Autodesk Fusion 360 part; units mm, degrees
(part 2 of 2)
sketch "Sketch10" plane through (0, 0, 0) normal (0, 0, 1) x (-1, 0, 0)
  line L0 (-14.3967, 6.981) -> (-3.4714, 1.9873)
  arc A0 (-3.4714, 1.9873) -> (-4, 0.0153) centre (0, 0) ccw
  line L1 (-4, 0.0153) -> (-12.1678, 3.0017)
  arc A1 (-14.3967, 6.981) -> (-12.1678, 3.0017) centre (-10.9658, 6.2889) ccw
  line L2 (-11.0881, -11.5349) -> (-2.9627, -2.6874)
  arc A2 (-2.9627, -2.6874) -> (-1.2506, -3.7995) centre (0, 0) ccw
  line L3 (-1.2506, -3.7995) -> (-6.6149, -10.6446)
  arc A3 (-11.0881, -11.5349) -> (-6.6149, -10.6446) centre (-9.3697, -8.4858) ccw
  line L4 (2.1904, 15.8494) -> (0.8173, 3.9156)
  arc A4 (0.8173, 3.9156) -> (-1.2215, 3.8089) centre (0, 0) ccw
  line L5 (-1.2215, 3.8089) -> (-0.9052, 12.4998)
  arc A5 (2.1904, 15.8494) -> (-0.9052, 12.4998) centre (2.5925, 12.3725) ccw
  line L6 (7.5439, -14.1099) -> (1.6404, -3.6482)
  arc A6 (1.6404, -3.6482) -> (3.2271, -2.3635) centre (0, 0) ccw
  line L7 (3.2271, -2.3635) -> (8.0795, -9.5805)
  arc A7 (7.5439, -14.1099) -> (8.0795, -9.5805) centre (5.175, -11.5334) ccw
  line L8 (15.7505, 2.8145) -> (3.9765, 0.4327)
  arc A8 (3.9765, 0.4327) -> (3.245, 2.3388) centre (0, 0) ccw
  line L9 (3.245, 2.3388) -> (11.6083, 4.7236)
  arc A9 (15.7505, 2.8145) -> (11.6083, 4.7236) centre (12.5681, 1.3577) ccw
  circle A10 centre (0, 0) radius 1.45
  line L10 (-3.1065, -11.6591) -> (-2.9735, -11.007)
  line L11 (-2.9735, -11.007) -> (-2.7469, -11.007)
  line L12 (-2.7469, -11.007) -> (-2.6562, -11.3012)
  line L13 (-2.6562, -11.3012) -> (-3.1065, -11.6591)
  line L14 (-11.5688, -0.9661) -> (-12.0485, -0.6484)
  line L15 (-12.0485, -0.6484) -> (-11.3871, -0.5734)
  line L16 (-11.3871, -0.5734) -> (-11.3171, -0.7889)
  line L17 (-11.3171, -0.7889) -> (-11.5688, -0.9661)
  line L18 (-4.4938, 10.7041) -> (-4.3398, 11.2584)
  line L19 (-4.3398, 11.2584) -> (-4.0641, 10.6526)
  line L20 (-4.0641, 10.6526) -> (-4.2475, 10.5194)
  line L21 (-4.2475, 10.5194) -> (-4.4938, 10.7041)
  line L22 (8.7916, 7.5816) -> (9.3663, 7.6065)
  line L23 (9.3663, 7.6065) -> (8.8753, 7.157)
  line L24 (8.8753, 7.157) -> (8.692, 7.2903)
  line L25 (8.692, 7.2903) -> (8.7916, 7.5816)
  line L26 (9.9272, -6.0184) -> (10.1285, -6.5574)
  line L27 (10.1285, -6.5574) -> (9.5494, -6.2293)
  line L28 (9.5494, -6.2293) -> (9.6194, -6.0137)
  line L29 (9.6194, -6.0137) -> (9.9272, -6.0184)
  line L30 (-2.5, -10.9982) -> (-2.7496, -10.5143)
  line L31 (-2.7496, -10.5143) -> (-2.3084, -9.7293)
  line L32 (-2.3084, -9.7293) -> (-1.3334, -9.8678)
  line L33 (-1.3334, -9.8678) -> (-1.5082, -10.5143)
  line L34 (-1.5082, -10.5143) -> (-2.1168, -10.9982)
  line L35 (-2.1168, -10.9982) -> (-2.5, -10.9982)
  line L36 (-9.7969, -1.7812) -> (-10.4658, -1.8148)
  line L37 (-10.4658, -1.8148) -> (-11.114, -1.3854)
  line L38 (-11.114, -1.3854) -> (-11.2324, -1.021)
  line L39 (-11.2324, -1.021) -> (-10.8494, -0.634)
  line L40 (-10.8494, -0.634) -> (-9.9664, -0.8111)
  line L41 (-9.9664, -0.8111) -> (-9.7969, -1.7812)
  line L42 (-4.7214, 8.767) -> (-4.9601, 9.3928)
  line L43 (-4.9601, 9.3928) -> (-4.752, 10.1419)
  line L44 (-4.752, 10.1419) -> (-4.442, 10.3672)
  line L45 (-4.442, 10.3672) -> (-3.9557, 10.1225)
  line L46 (-3.9557, 10.1225) -> (-3.8512, 9.228)
  line L47 (-3.8512, 9.228) -> (-4.7214, 8.767)
  line L48 (6.8789, 7.1995) -> (7.4003, 7.6198)
  line L49 (7.4003, 7.6198) -> (8.1771, 7.6535)
  line L50 (8.1771, 7.6535) -> (8.4871, 7.4282)
  line L51 (8.4871, 7.4282) -> (8.4047, 6.8901)
  line L52 (8.4047, 6.8901) -> (7.5863, 6.5143)
  line L53 (7.5863, 6.5143) -> (6.8789, 7.1995)
  line L54 (8.9728, -4.3175) -> (9.5337, -4.6835)
  line L55 (9.5337, -4.6835) -> (9.8057, -5.4118)
  line L56 (9.8057, -5.4118) -> (9.6873, -5.7763)
  line L57 (9.6873, -5.7763) -> (9.1501, -5.8642)
  line L58 (9.1501, -5.8642) -> (8.5397, -5.2019)
  line L59 (8.5397, -5.2019) -> (8.9728, -4.3175)
  line L60 (-5.9663, -3.6633) -> (-7.4659, -4.5288)
  line L61 (-7.4659, -4.5288) -> (-8.4085, -3.5945)
  line L62 (-8.4085, -3.5945) -> (-8.393, -1.6756)
  line L63 (-8.393, -1.6756) -> (-6.9045, -0.8166)
  line L64 (-6.9045, -0.8166) -> (-5.7063, -1.8541)
  line L65 (-5.7063, -1.8541) -> (-5.9663, -3.6633)
  line L66 (-5.3277, 4.5422) -> (-6.6142, 5.7011)
  line L67 (-6.6142, 5.7011) -> (-6.0169, 6.8862)
  line L68 (-6.0169, 6.8862) -> (-4.1872, 7.4644)
  line L69 (-4.1872, 7.4644) -> (-2.9103, 6.3142)
  line L70 (-2.9103, 6.3142) -> (-3.5267, 4.8541)
  line L71 (-3.5267, 4.8541) -> (-5.3277, 4.5422)
  line L72 (6.9189, -5.2232) -> (7.2026, -4.6437)
  line L73 (7.2026, -4.6437) -> (7.9541, -5.0117)
  line L74 (7.9541, -5.0117) -> (7.869, -5.7717)
  line L75 (7.869, -5.7717) -> (7.2097, -5.6979)
  line L76 (7.2097, -5.6979) -> (6.9189, -5.2232)
  line L77 (7.1056, 4.9662) -> (6.6422, 5.4151)
  line L78 (6.6422, 5.4151) -> (7.2243, 6.0161)
  line L79 (7.2243, 6.0161) -> (7.9209, 5.7004)
  line L80 (7.9209, 5.7004) -> (7.6469, 5.0961)
  line L81 (7.6469, 5.0961) -> (7.1056, 4.9662)
  line L82 (-2.5274, 8.2925) -> (-3.0976, 7.9904)
  line L83 (-3.0976, 7.9904) -> (-3.4892, 8.7298)
  line L84 (-3.4892, 8.7298) -> (-2.9737, 9.2947)
  line L85 (-2.9737, 9.2947) -> (-2.4836, 8.8474)
  line L86 (-2.4836, 8.8474) -> (-2.5274, 8.2925)
  line L87 (-8.6676, 0.1588) -> (-8.5566, -0.4768)
  line L88 (-8.5566, -0.4768) -> (-9.3808, -0.6208)
  line L89 (-9.3808, -0.6208) -> (-9.7587, 0.0441)
  line L90 (-9.7587, 0.0441) -> (-9.1819, 0.3719)
  line L91 (-9.1819, 0.3719) -> (-8.6676, 0.1588)
  line L92 (-2.8295, -8.1943) -> (-2.1907, -8.2851)
  line L93 (-2.1907, -8.2851) -> (-2.3084, -9.1135)
  line L94 (-2.3084, -9.1135) -> (-3.0575, -9.2674)
  line L95 (-3.0575, -9.2674) -> (-3.1911, -8.6176)
  line L96 (-3.1911, -8.6176) -> (-2.8295, -8.1943)
  line L97 (8.133, -6.2409) -> (8.0476, -6.0122)
  line L98 (8.0476, -6.0122) -> (8.138, -5.8407)
  line L99 (8.138, -5.8407) -> (8.3643, -5.9142)
  line L100 (8.3643, -5.9142) -> (8.5351, -6.3715)
  line L101 (8.5351, -6.3715) -> (8.133, -6.2409)
  line L102 (8.4487, 5.8064) -> (8.2048, 5.7959)
  line L103 (8.2048, 5.7959) -> (8.0696, 5.9348)
  line L104 (8.0696, 5.9348) -> (8.2095, 6.1273)
  line L105 (8.2095, 6.1273) -> (8.6972, 6.1485)
  line L106 (8.6972, 6.1485) -> (8.4487, 5.8064)
  line L107 (-2.9115, 9.8295) -> (-2.9768, 9.5943)
  line L108 (-2.9768, 9.5943) -> (-3.1507, 9.5086)
  line L109 (-3.1507, 9.5086) -> (-3.2906, 9.7011)
  line L110 (-3.2906, 9.7011) -> (-3.16, 10.1715)
  line L111 (-3.16, 10.1715) -> (-2.9115, 9.8295)
  line L112 (-10.2481, 0.2685) -> (-10.0446, 0.1337)
  line L113 (-10.0446, 0.1337) -> (-10.0168, -0.0582)
  line L114 (-10.0168, -0.0582) -> (-10.2432, -0.1317)
  line L115 (-10.2432, -0.1317) -> (-10.6502, 0.1379)
  line L116 (-10.6502, 0.1379) -> (-10.2481, 0.2685)
  line L117 (-3.4222, -10.0863) -> (-3.4222, -9.6635)
  line L118 (-3.4222, -9.6635) -> (-3.2311, -9.5116)
  line L119 (-3.2311, -9.5116) -> (-3.04, -9.5445)
  line L120 (-3.04, -9.5445) -> (-3.04, -9.7825)
  line L121 (-3.04, -9.7825) -> (-3.4222, -10.0863)
  line L122 (-0.9521, -12.3007) -> (-0.9521, -11.7519)
  line L123 (-0.9521, -11.7519) -> (-0.7677, -11.7519)
  line L124 (-0.7677, -11.7519) -> (-0.5833, -11.869)
  line L125 (-0.5833, -11.869) -> (-0.9521, -12.3007)
  line L126 (-11.414, -2.9014) -> (-11.4683, -3.113)
  line L127 (-11.4683, -3.113) -> (-11.9929, -2.8956)
  line L128 (-11.9929, -2.8956) -> (-11.471, -2.726)
  line L129 (-11.471, -2.726) -> (-11.414, -2.9014)
  line L130 (-6.2865, 9.9588) -> (-6.5045, 9.9451)
  line L131 (-6.5045, 9.9451) -> (-6.4599, 10.5111)
  line L132 (-6.4599, 10.5111) -> (-6.1373, 10.0672)
  line L133 (-6.1373, 10.0672) -> (-6.2865, 9.9588)
  line L134 (7.5287, 9.0563) -> (7.4483, 9.2594)
  line L135 (7.4483, 9.2594) -> (8.0005, 9.3919)
  line L136 (8.0005, 9.3919) -> (7.6779, 8.9479)
  line L137 (7.6779, 8.9479) -> (7.5287, 9.0563)
  line L138 (10.9395, -4.3617) -> (11.1078, -4.2225)
  line L139 (11.1078, -4.2225) -> (11.4045, -4.7067)
  line L140 (11.4045, -4.7067) -> (10.8825, -4.5371)
  line L141 (10.8825, -4.5371) -> (10.9395, -4.3617)
  line L142 (-0.7484, -11.4996) -> (-0.7484, -10.5143)
  line L143 (-0.7484, -10.5143) -> (-0.1481, -10.0371)
  line L144 (-0.1481, -10.0371) -> (0.4215, -10.1911)
  line L145 (0.4215, -10.1911) -> (0.4215, -10.8376)
  line L146 (0.4215, -10.8376) -> (-0.1481, -11.4996)
  line L147 (-0.1481, -11.4996) -> (-0.7484, -11.4996)
  line L148 (-9.562, -3.5501) -> (-10.1769, -3.7499)
  line L149 (-10.1769, -3.7499) -> (-10.9825, -3.4127)
  line L150 (-10.9825, -3.4127) -> (-11.168, -2.8417)
  line L151 (-11.168, -2.8417) -> (-10.231, -2.5373)
  line L152 (-10.231, -2.5373) -> (-9.5916, -2.9608)
  line L153 (-9.5916, -2.9608) -> (-9.562, -3.5501)
  line L154 (-6.3312, 7.997) -> (-6.7112, 8.5201)
  line L155 (-6.7112, 8.5201) -> (-6.6395, 9.3904)
  line L156 (-6.6395, 9.3904) -> (-6.1538, 9.7433)
  line L157 (-6.1538, 9.7433) -> (-5.5747, 8.9462)
  line L158 (-5.5747, 8.9462) -> (-5.7799, 8.2073)
  line L159 (-5.7799, 8.2073) -> (-6.3312, 7.997)
  line L160 (5.6492, 8.4925) -> (6.0292, 9.0156)
  line L161 (6.0292, 9.0156) -> (6.8791, 9.2163)
  line L162 (6.8791, 9.2163) -> (7.3648, 8.8634)
  line L163 (7.3648, 8.8634) -> (6.7857, 8.0664)
  line L164 (6.7857, 8.0664) -> (6.0195, 8.0332)
  line L165 (6.0195, 8.0332) -> (5.6492, 8.4925)
  line L166 (9.8225, -2.7484) -> (10.4374, -2.9482)
  line L167 (10.4374, -2.9482) -> (10.891, -3.6944)
  line L168 (10.891, -3.6944) -> (10.7054, -4.2654)
  line L169 (10.7054, -4.2654) -> (9.7685, -3.9609)
  line L170 (9.7685, -3.9609) -> (9.5001, -3.2425)
  line L171 (9.5001, -3.2425) -> (9.8225, -2.7484)
  line L172 (0.8202, -9.1077) -> (-1, -8.5)
  line L173 (-1, -8.5) -> (-1.357, -6.8189)
  line L174 (-1.357, -6.8189) -> (0, -6)
  line L175 (0, -6) -> (1.6404, -6.8063)
  line L176 (1.6404, -6.8063) -> (2, -8.5)
  line L177 (2, -8.5) -> (0.8202, -9.1077)
  line L178 (2.6736, 6.4706) -> (3.3781, 8.0522)
  line L179 (3.3781, 8.0522) -> (4.6898, 7.8504)
  line L180 (4.6898, 7.8504) -> (5.8052, 6.2889)
  line L181 (5.8052, 6.2889) -> (5.1059, 4.719)
  line L182 (5.1059, 4.719) -> (3.5267, 4.8541)
  line L183 (3.5267, 4.8541) -> (2.6736, 6.4706)
  line L184 (6.9801, -0.5432) -> (8.702, -0.7245)
  line L185 (8.702, -0.7245) -> (8.9154, -2.0344)
  line L186 (8.9154, -2.0344) -> (7.775, -3.5777)
  line L187 (7.775, -3.5777) -> (6.0658, -3.3977)
  line L188 (6.0658, -3.3977) -> (5.7063, -1.8541)
  line L189 (5.7063, -1.8541) -> (6.9801, -0.5432)
  line L190 (10.7785, -1.3057) -> (11.2993, -2.1887)
  line L191 (11.2993, -2.1887) -> (10.2999, -2.0834)
  line L192 (10.2999, -2.0834) -> (10.0348, -1.8876)
  line L193 (10.0348, -1.8876) -> (9.7957, -1.1372)
  line L194 (9.7957, -1.1372) -> (10.4141, -1.0365)
  line L195 (10.4141, -1.0365) -> (10.7785, -1.3057)
  line L196 (4.5725, 9.8475) -> (5.5732, 10.0699)
  line L197 (5.5732, 10.0699) -> (5.1643, 9.1519)
  line L198 (5.1643, 9.1519) -> (4.8961, 8.9604)
  line L199 (4.8961, 8.9604) -> (4.1086, 8.9648)
  line L200 (4.1086, 8.9648) -> (4.2039, 9.5842)
  line L201 (4.2039, 9.5842) -> (4.5725, 9.8475)
  line L202 (-7.9525, 7.3918) -> (-7.8548, 8.4122)
  line L203 (-7.8548, 8.4122) -> (-7.1081, 7.7396)
  line L204 (-7.1081, 7.7396) -> (-7.0089, 7.4254)
  line L205 (-7.0089, 7.4254) -> (-7.2564, 6.6778)
  line L206 (-7.2564, 6.6778) -> (-7.816, 6.9598)
  line L207 (-7.816, 6.9598) -> (-7.9525, 7.3918)
  line L208 (-9.4874, -5.2791) -> (-10.4278, -4.8709)
  line L209 (-10.4278, -4.8709) -> (-9.5574, -4.3686)
  line L210 (-9.5574, -4.3686) -> (-9.2278, -4.3712)
  line L211 (-9.2278, -4.3712) -> (-8.5933, -4.8377)
  line L212 (-8.5933, -4.8377) -> (-9.0344, -5.2828)
  line L213 (-9.0344, -5.2828) -> (-9.4874, -5.2791)
  line L214 (1.4101, -11.4226) -> (1.2014, -10.4396)
  line L215 (1.2014, -10.4396) -> (1.3057, -10.127)
  line L216 (1.3057, -10.127) -> (1.9455, -9.6677)
  line L217 (1.9455, -9.6677) -> (2.2324, -10.2247)
  line L218 (2.2324, -10.2247) -> (2.0889, -10.6544)
  line L219 (2.0889, -10.6544) -> (1.4101, -11.4226)
  line L220 (11.7371, -2.286) -> (12.0169, -2.7428)
  line L221 (12.0169, -2.7428) -> (11.4775, -2.4787)
  line L222 (11.4775, -2.4787) -> (11.5012, -2.2543)
  line L223 (11.5012, -2.2543) -> (11.7371, -2.286)
  line L224 (5.801, 10.4562) -> (6.322, 10.5812)
  line L225 (6.322, 10.5812) -> (5.9041, 10.1498)
  line L226 (5.9041, 10.1498) -> (5.698, 10.2417)
  line L227 (5.698, 10.2417) -> (5.801, 10.4562)
  line L228 (-8.1518, 8.7483) -> (-8.1097, 9.2824)
  line L229 (-8.1097, 9.2824) -> (-7.8286, 8.7516)
  line L230 (-7.8286, 8.7516) -> (-7.9796, 8.584)
  line L231 (-7.9796, 8.584) -> (-8.1518, 8.7483)
  line L232 (-10.8391, -5.0495) -> (-11.3341, -4.8444)
  line L233 (-11.3341, -4.8444) -> (-10.7425, -4.741)
  line L234 (-10.7425, -4.741) -> (-10.6297, -4.9365)
  line L235 (-10.6297, -4.9365) -> (-10.8391, -5.0495)
  line L236 (1.1049, -12.2764) -> (1.1894, -11.6818)
  line L237 (1.1894, -11.6818) -> (1.4101, -11.6349)
  line L238 (1.4101, -11.6349) -> (1.4529, -11.869)
  line L239 (1.4529, -11.869) -> (1.1049, -12.2764)
  circle A11 centre (0, 0) radius 19
